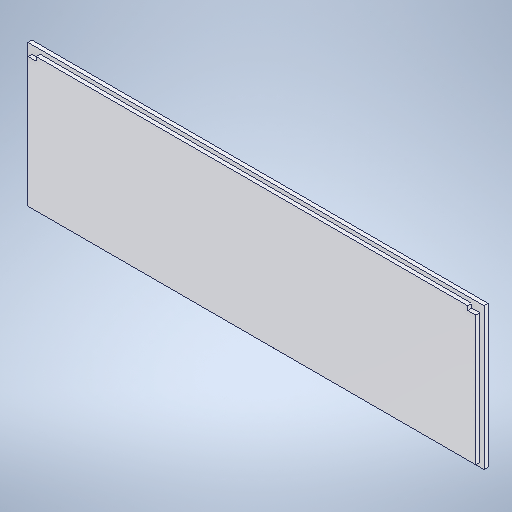
# Autodesk Inventor part: back
Saved by Autodesk Inventor 2025 (Build 290162000, 162)
## iProperties
Created: 2025-05-20
Part Number: back
Material: Generic
Document SubType Name: Modeling
Designer: ethan
Density: 1 g/cm^3
Appearance: PTFE
Author: ethan
Autodesk Inventor part; units mm, degrees
ref_plane "YZ Plane" through (0, 0, 0) normal (1, 0, 0) x (0, 1, 0)
ref_plane "XZ Plane" through (0, 0, 0) normal (0, 1, 0) x (-1, 0, 0)
ref_plane "XY Plane" through (0, 0, 0) normal (0, 0, 1) x (1, 0, 0)
sketch "Sketch1" plane through (0, 0, 0) normal (0, 0, 1) x (1, 0, 0)
  line L0 (0, 0) -> (224.6, 0)
  line L1 (224.6, 0) -> (224.6, 69.85)
  line L2 (224.6, 69.85) -> (0, 69.85)
  line L3 (0, 69.85) -> (0, 0)
  dimension "d0" = 224.6
  dimension "d1" = 69.85
  constraints: 8 end point, 2 parallel, 1 horizontal, 1 perpendicular
  measures "d0" distance of L2.end L1.end
  measures "d1" distance of L1.end L0.end
extrude "Extrusion1" add sketch "Sketch1" along normal blind 2
sketch "Sketch2" plane through (0, 0, 2) normal (0, 0, 1) x (1, 0, 0)
  line L0 (224.6, 0) -> (224.6, 69.85) projected
  line L1 (224.6, 69.85) -> (0, 69.85) projected
  line L2 (0, 69.85) -> (0, 0) projected
  line L3 (0, 0) -> (224.6, 0) projected
  line L4 (2, 67.85) -> (222.6, 67.85)
  line L5 (222.6, 67.85) -> (222.6, 2)
  line L6 (222.6, 2) -> (2, 2)
  line L7 (2, 2) -> (2, 67.85)
  dimension "d4" = 2
  constraints: 8 end point, 3 other
  measures "d4" distance between parallel lines of L1 L4
extrude "Extrusion2" add sketch "Sketch2" along normal blind 2 contours L4 L5 L6 L7
sketch "Sketch3" plane through (0, 0, 4) normal (0, 0, 1) x (1, 0, 0)
  line L0 (2, 2) -> (222.6, 2) construction
  line L1 (222.6, 2) -> (222.6, 67.85) construction
  line L2 (222.6, 67.85) -> (2, 67.85) construction
  line L3 (2, 67.85) -> (2, 2) construction
  line L4 (2, 67.85) -> (6, 67.85)
  line L5 (6, 67.85) -> (6, 65.85)
  line L6 (6, 65.85) -> (2, 65.85)
  line L7 (2, 65.85) -> (2, 67.85)
  line L8 (222.6, 67.85) -> (218.6, 67.85)
  line L9 (218.6, 67.85) -> (218.6, 65.85)
  line L10 (218.6, 65.85) -> (222.6, 65.85)
  line L11 (222.6, 65.85) -> (222.6, 67.85)
  point P0 (0, 0)
  dimension "d7" = 4
  dimension "d8" = 2
  dimension "d9" = 4
  dimension "d10" = 2
  constraints: 16 end point, 4 parallel, 2 horizontal, 2 perpendicular
  measures "d7" distance of L5.end L6.end
  measures "d8" distance of L4.end L5.end
  measures "d9" distance of L10.end L9.end
  measures "d10" distance of L9.end L8.end
extrude "Extrusion3" cut sketch "Sketch3" against normal blind 2
body "Solid1"
